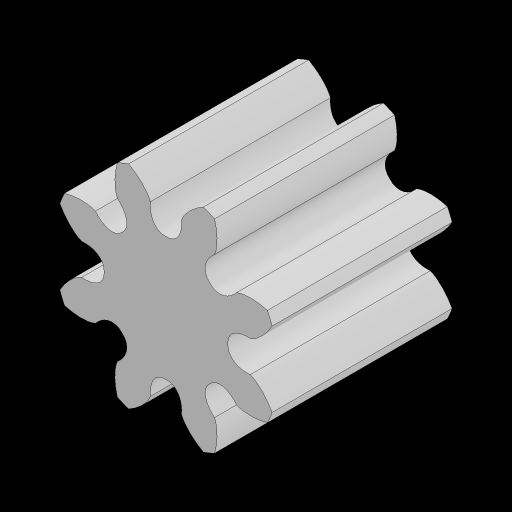
# Autodesk Inventor part: Servo Gear
Saved by Autodesk Inventor 2023.2 (Build 272271030, 271C)
## iProperties
Created: 2023-11-08
Part Number: Servo Gear
Material: Generic
Document SubType Name: Modeling
Designer: robpl
Density: 1 g/cm^3
Appearance: Default
Author: robpl
Autodesk Inventor part; units mm, degrees
ref_plane "YZ Plane" through (0, 0, 0) normal (1, 0, 0) x (0, 1, 0)
ref_plane "XZ Plane" through (0, 0, 0) normal (0, 1, 0) x (-1, 0, 0)
ref_plane "XY Plane" through (0, 0, 0) normal (0, 0, 1) x (1, 0, 0)
sketch "Sketch1" plane through (0, 0, 0) normal (0, 0, 1) x (1, 0, 0)
  spline S0 degree 3 poles (-2.0759, 5.8952) (-2.0129, 5.8587) (-1.8871, 5.7857) (-1.7067, 5.6627) (-1.5336, 5.5298) (-1.3698, 5.3855) (-1.2169, 5.2296) (-1.1008, 5.0894) (-1.0166, 4.9708) (-0.9588, 4.8782) (-0.9063, 4.7824) (-0.8792, 4.7149) (-0.8657, 4.6811) knots 0 0 0 0 0.021814 0.043629 0.065444 0.087257 0.10907 0.13088 0.141788 0.152695 0.163602 0.174505 0.174505 0.174505 0.174505
  spline S1 degree 3 poles (-0.8657, 4.6811) (-0.8686, 4.645) (-0.8745, 4.5727) (-0.8747, 4.4638) (-0.8681, 4.3553) (-0.856, 4.2471) (-0.8344, 4.1405) (-0.8059, 4.0354) (-0.7666, 3.9338) (-0.7187, 3.8361) (-0.6601, 3.7442) (-0.5905, 3.6604) (-0.5105, 3.5863) (-0.4204, 3.5247) (-0.322, 3.4775) (-0.2346, 3.4523) (-0.1631, 3.4403) (-0.0906, 3.4359) (0, 3.4385) (0.0906, 3.4359) (0.1631, 3.4403) (0.2346, 3.4523) (0.322, 3.4775) (0.4204, 3.5247) (0.5105, 3.5863) (0.5905, 3.6604) (0.6601, 3.7442) (0.7187, 3.8361) (0.7666, 3.9338) (0.8059, 4.0354) (0.8344, 4.1405) (0.856, 4.2471) (0.8681, 4.3553) (0.8747, 4.4638) (0.8745, 4.5727) (0.8686, 4.645) (0.8657, 4.6811) knots 0 0 0 0 0.010873 0.021747 0.032621 0.043493 0.054365 0.065238 0.07611 0.086978 0.09785 0.10872 0.119589 0.130456 0.141322 0.152184 0.157624 0.163058 0.173931 0.184805 0.190238 0.195678 0.20654 0.217407 0.228273 0.239142 0.250013 0.260884 0.271753 0.282624 0.293497 0.304369 0.315242 0.326115 0.33699 0.347862 0.347862 0.347862 0.347862
  spline S2 degree 3 poles (0.8657, 4.6811) (0.8792, 4.7149) (0.9063, 4.7824) (0.9588, 4.8782) (1.0166, 4.9708) (1.1008, 5.0894) (1.2169, 5.2296) (1.3698, 5.3855) (1.5336, 5.5298) (1.7067, 5.6627) (1.8871, 5.7857) (2.0129, 5.8587) (2.0759, 5.8952) knots 0 0 0 0 0.010904 0.02181 0.032717 0.043625 0.065435 0.087248 0.109062 0.130876 0.152691 0.174505 0.174505 0.174505 0.174505
  circle A0 centre (0, 0) radius 3.4375 construction
  circle A1 centre (0, 0) radius 4.6985 construction
  circle A2 centre (0, 0) radius 5 construction
  circle A3 centre (0, 0) radius 6.25
  point P0 (-1.8885, 5.7835)
  point P1 (-1.7079, 5.6611)
  point P2 (-1.5351, 5.5279)
  point P3 (-1.3716, 5.3836)
  point P4 (-1.2192, 5.2275)
  point P5 (-1.0805, 5.0592)
  point P6 (-1.0175, 4.9702)
  point P7 (-0.9597, 4.8777)
  point P8 (-0.9083, 4.7815)
  point P9 (-0.8731, 4.5726)
  point P10 (-0.8735, 4.4639)
  point P11 (-0.8672, 4.3553)
  point P12 (-0.8544, 4.2474)
  point P13 (-0.8332, 4.1407)
  point P14 (-0.8041, 4.036)
  point P15 (-0.7652, 3.9345)
  point P16 (-0.7169, 3.8371)
  point P17 (-0.6582, 3.7456)
  point P18 (-0.5887, 3.662)
  point P19 (-0.5088, 3.5884)
  point P20 (-0.419, 3.5271)
  point P21 (-0.3209, 3.4803)
  point P22 (-0.2166, 3.45)
  point P23 (-0.1629, 3.4412)
  point P24 (-0.1087, 3.4375)
  point P25 (0, 3.4375)
  point P26 (0.1087, 3.4375)
  point P27 (0.1629, 3.4412)
  point P28 (0.2166, 3.45)
  point P29 (0.3209, 3.4803)
  point P30 (0.419, 3.5271)
  point P31 (0.5088, 3.5884)
  point P32 (0.5887, 3.662)
  point P33 (0.6582, 3.7456)
  point P34 (0.7169, 3.8371)
  point P35 (0.7652, 3.9345)
  point P36 (0.8041, 4.036)
  point P37 (0.8332, 4.1407)
  point P38 (0.8544, 4.2474)
  point P39 (0.8672, 4.3553)
  point P40 (0.8735, 4.4639)
  point P41 (0.8731, 4.5726)
  point P42 (0.9083, 4.7815)
  point P43 (0.9597, 4.8777)
  point P44 (1.0175, 4.9702)
  point P45 (1.0805, 5.0592)
  point P46 (1.2192, 5.2275)
  point P47 (1.3716, 5.3836)
  point P48 (1.5351, 5.5279)
  point P49 (1.7079, 5.6611)
  point P50 (1.8885, 5.7835)
  constraints: 4 centre point, 2 point on circle, 117 other
extrude "Extrusion1" add sketch "Sketch1" against normal blind 10
extrude "Extrusion2" cut sketch "Sketch1" against normal through all contours A3 S2 S1 S0 picked at (0.2443, 5.3779)
pattern_circular "Circular Pattern1" count 8 over 360 about axis through (0, 0, 0) along (0, 0, -1) of "Extrusion2"
equation "\"Module\" = 1.25"
equation "\"PressureAngle\" = 20deg"
equation "\"UnitProfileClearance\" = 0.25"
equation "\"UnitRoundRadius\" = 0.35"
equation "\"HeadDiameter\" = 12.5"
equation "\"RootDiameter\" = 6.875"
equation "\"BaseDiameter\" = 9.39693"
equation "\"HelixAngle\" = 0"
equation "\"UnitCorrection\" = 0"
equation "\"UnitAddendumModification\" = 0"
equation "\"CircularPitch\" = 3.926991"
equation "\"UnitBacklashShift\" = 0"
equation "\"TotalToolShift\" = 0"
equation "\"IsInternal\" = 0"
body "Solid1"
